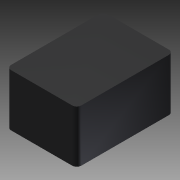
# Autodesk Inventor part: Cam.Silicon.back
Saved by Autodesk Inventor 2011 (Build 150239000, 239)
## iProperties
Created: 2011-03-27
Part Number: Cam.Silicon.back
Document SubType Name: Modeling
Designer: Rob
Density: 1.25 g/cm^3
Material: Silicone
Mass: 29.0927 g
Surface Area: 236.315 cm^2
Volume: 23.2741 cm^3
Author: Rob
Autodesk Inventor part; units mm, degrees
ref_plane "YZ Plane" through (0, 0, 0) normal (1, 0, 0) x (0, 1, 0)
ref_plane "XZ Plane" through (0, 0, 0) normal (0, 1, 0) x (-1, 0, 0)
ref_plane "XY Plane" through (0, 0, 0) normal (0, 0, 1) x (1, 0, 0)
sketch "Sketch1" plane through (0, 0, 0) normal (0, 0, 1) x (1, 0, 0)
  line L0 (-21.1, 29.81) -> (21.1, 29.81)
  line L1 (21.1, 29.81) -> (21.1, -29.81)
  line L2 (21.1, -29.81) -> (-21.1, -29.81)
  line L3 (-21.1, -29.81) -> (-21.1, 29.81)
  line L4 (0, 0) -> (0, 68.2086)
  line L5 (0, 0) -> (53.7664, 0)
  line L6 (-21.1, 29.81) -> (21.1, 29.81)
  line L7 (21.1, 29.81) -> (21.1, -29.81)
  line L8 (21.1, -29.81) -> (-21.1, -29.81)
  line L9 (-21.1, -29.81) -> (-21.1, 29.81)
  line L10 (0, 0) -> (0, 68.2086)
  line L11 (0, 0) -> (54.462, 0)
  line L12 (-23.1, 31.81) -> (23.1, 31.81)
  line L13 (23.1, 31.81) -> (23.1, -31.81)
  line L14 (23.1, -31.81) -> (-23.1, -31.81)
  line L15 (-23.1, -31.81) -> (-23.1, 31.81)
  line L16 (-26.1, 34.81) -> (26.1, 34.81)
  line L17 (26.1, 34.81) -> (26.1, -34.81)
  line L18 (26.1, -34.81) -> (-26.1, -34.81)
  line L19 (-26.1, -34.81) -> (-26.1, 34.81)
  dimension "d0" = 59.62
  dimension "d1" = 42.2
  dimension "d2" = 59.62
  dimension "d3" = 42.2
  dimension "d4" = 2
  dimension "d5" = 2
  dimension "d6" = 0
  dimension "d7" = 3
  dimension "d8" = 3
  constraints: 40 end point, 10 parallel, 6 perpendicular, 4 horizontal, 8 other
  measures "d0" distance between parallel lines of L2 L0
  measures "d1" distance between parallel lines of L1 L3
  measures "d2" distance between parallel lines of L8 L6
  measures "d3" distance between parallel lines of L7 L9
  measures "d4" distance between parallel lines of L6 L12
  measures "d5" distance between parallel lines of L15 L9
  measures "d6" distance of point (0, 0) L10.start
  measures "d7" distance between parallel lines of L12 L16
  measures "d8" distance between parallel lines of L17 L13
extrude "Extrusion1" add sketch "Sketch1" along normal blind 30.3 contours L3 L2 L1 L5 L13 L14 L15 L12 L4 L0 | L4 L12 L13 L5 L1 L0
sketch "Sketch2" plane through (0, 0, 30.3) normal (0, 0, 1) x (1, 0, 0)
  line L0 (-23.1, -31.81) -> (23.1, -31.81)
  line L1 (23.1, -31.81) -> (23.1, 31.81)
  line L2 (23.1, 31.81) -> (-23.1, 31.81)
  line L3 (-23.1, 31.81) -> (-23.1, -31.81)
  point P0 (0, 0)
  constraints: 8 end point, 2 parallel, 1 horizontal, 1 perpendicular
extrude "Extrusion2" add sketch "Sketch2" along normal blind 2
sketch "Sketch3" plane through (0, 0, 0) normal (0, 0, -1) x (-1, 0, 0)
  line L0 (-23.1, -31.81) -> (23.1, -31.81) projected
  line L1 (23.1, -31.81) -> (23.1, 31.81) projected
  line L2 (23.1, 31.81) -> (-23.1, 31.81) projected
  line L3 (-23.1, 31.81) -> (-23.1, -31.81) projected
  circle A0 centre (-3.92, 14.54) radius 10.07
  line L4 (21.1, 29.81) -> (21.1, -29.81)
  line L5 (-21.1, 29.81) -> (21.1, 29.81)
  line L6 (-21.1, -29.81) -> (-21.1, 29.81)
  line L7 (21.1, -29.81) -> (-21.1, -29.81)
  point P0 (0, 0)
  point P1 (0, 0)
  constraints: 8 end point, 1 centre point
extrude "Extrusion3" add sketch "Sketch3" along normal blind 2 contours L3 L2 L1 L0 | L4 L7 L6 L5
fillet "Fillet3" radius 3 4 edges at (-23.1, -31.81, 15.15) (-23.1, 31.81, 15.15) (23.1, -31.81, 15.15) (23.1, 31.81, 15.15)
equation "\"d5\" = d4"
equation "\"d8\" = d7"
body "Solid1"
